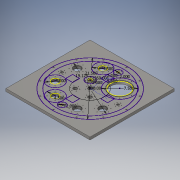
# Autodesk Inventor part: Top Plate
Saved by Autodesk Inventor 2018 (Build 220112000, 112)
## iProperties
Created: 2018-08-07
Part Number: Top Plate
Material: Stainless Steel, Austenitic
Document SubType Name: Modeling
Designer: freyja
Density: 8 g/cm^3
Appearance: Semi-Polished
Mass: 52241 g
Surface Area: 7917.75 cm^2
Volume: 6530.12 cm^3
Author: freyja
Autodesk Inventor part; units mm, degrees
ref_plane "YZ Plane" through (0, 0, 0) normal (1, 0, 0) x (0, 1, 0)
ref_plane "XZ Plane" through (0, 0, 0) normal (0, 1, 0) x (-1, 0, 0)
ref_plane "XY Plane" through (0, 0, 0) normal (0, 0, 1) x (1, 0, 0)
sketch "Sketch1" plane through (0, 0, 0) normal (0, 1, 0) x (-1, 0, 0)
  line L0 (304.8, 304.8) -> (-304.8, 304.8)
  line L1 (-304.8, 304.8) -> (-304.8, -304.8)
  line L2 (-304.8, -304.8) -> (304.8, -304.8)
  line L3 (304.8, -304.8) -> (304.8, 304.8)
  line L4 (304.8, 304.8) -> (-304.8, -304.8) construction
  line L5 (-304.8, 304.8) -> (304.8, -304.8) construction
  point P0 (0, 0)
  dimension "d0" = 609.6
  dimension "d1" = 609.6
  constraints: 12 end point, 2 midpoint, 2 parallel, 1 horizontal, 1 perpendicular
  measures "d0" distance of L2.end L1.end
  measures "d1" distance of L1.end L0.end
extrude "Extrusion1" add sketch "Sketch1" along normal blind 19.05
sketch "Sketch23" plane through (0, 19.05, 0) normal (0, 1, 0) x (1, 0, 0)
  circle A0 centre (0, 0) radius 273.05
  circle A1 centre (0, 0) radius 242.8875
  dimension "d167" = 546.1
  dimension "d168" = 485.775
  constraints: 2 centre point, 2 coincident
  measures "d167" diameter of A0
  measures "d168" diameter of A1
sketch "Sketch2" plane through (0, 19.05, 0) normal (0, 1, 0) x (1, 0, 0)
  line L0 (0, 0) -> (107.7631, 107.7631) construction
  line L1 (0, 0) -> (152.4, 0) construction
  circle A0 centre (107.7631, 107.7631) radius 118.745 construction
  circle A1 centre (107.7631, 107.7631) radius 66.675
  dimension "d4" = 152.4
  dimension "d5" = 45
  dimension "d6" = 237.49
  dimension "d7" = 133.35
  constraints: 4 end point, 2 centre point, 2 coincident, 1 equal length, 1 horizontal
  measures "d4" distance of L0.start L0.end
  measures "d5" angle of L1 L0
  measures "d6" diameter of A0
  measures "d7" diameter of A1
extrude "Extrusion2" cut sketch "Sketch2" against normal up to surface (19.05 mm away)
sketch "Sketch3" plane through (0, 19.05, 0) normal (0, 1, 0) x (1, 0, 0)
  circle A0 centre (107.7631, 107.7631) radius 66.675 projected
  line L0 (107.7631, 107.7631) -> (194.1231, 107.7631) construction
  line L1 (107.7631, 107.7631) -> (194.1231, 107.7631) construction
  line L2 (107.7631, 107.7631) -> (168.8288, 168.8288) construction
  line L3 (107.7631, 107.7631) -> (107.7631, 194.1231) construction
  line L4 (107.7631, 107.7631) -> (46.6973, 168.8288) construction
  line L5 (107.7631, 107.7631) -> (21.4031, 107.7631) construction
  line L6 (107.7631, 107.7631) -> (46.6973, 46.6973) construction
  line L7 (107.7631, 107.7631) -> (107.7631, 21.4031) construction
  line L8 (107.7631, 107.7631) -> (168.8288, 46.6973) construction
  point P0 (0, 0)
  dimension "d10" = 86.36
  dimension "d11" = 0
  dimension "d14" = 360
  constraints: 18 end point, 2 coincident, 2 horizontal, 1 collinear, 23 other
  measures "d10" distance of L0.start L0.end
  measures "d11" distance between parallel lines of L0 L1
hole "Hole1" at (194.1231, 19.05, -107.7631) at (168.8288, 19.05, -168.8288) at (107.7631, 19.05, -194.1231) at (46.6973, 19.05, -168.8288) at (21.4031, 19.05, -107.7631) at (46.6973, 19.05, -46.6973) at (107.7631, 19.05, -21.4031) at (168.8288, 19.05, -46.6973) direction (0, -1, 0) diameter 4.9784 depth 15.24 tip angle 118 thread size "1/4-20 UNC" class "2B" standard "ANSI Unified Screw Threads"
sketch "Sketch4" plane through (0, 19.05, 0) normal (0, 1, 0) x (1, 0, 0)
  line L0 (0, 0) -> (-172.6516, -80.5088) construction
  line L1 (0, 0) -> (190.5, 0) construction
  circle A0 centre (-172.6516, -80.5088) radius 26.289
  dimension "d23" = 190.5
  dimension "d24" = 205
  dimension "d25" = 52.578
  constraints: 4 end point, 1 centre point, 1 coincident, 1 equal length, 1 horizontal
  measures "d23" distance of L0.start L0.end
  measures "d25" diameter of A0
extrude "Extrusion3" cut sketch "Sketch4" against normal blind 2.54
sketch "Sketch5" plane through (-172.6516, 16.51, 80.5088) normal (0, 1, 0) x (1, 0, 0)
  circle A0 centre (0, 0) radius 26.289 projected
  circle A1 centre (0, 0) radius 24.13
  point P0 (172.6516, 80.5088)
  dimension "d28" = 48.26
  constraints: 1 centre point, 1 coincident
  measures "d28" diameter of A1
extrude "Extrusion4" cut sketch "Sketch5" against normal up to surface (16.51 mm away) contours A1
sketch "Sketch6" plane through (0, 19.05, 0) normal (0, 1, 0) x (1, 0, 0)
  circle A0 centre (-172.6516, -80.5088) radius 24.13 construction
  line L0 (-172.6516, -80.5088) -> (-131.3766, -80.5088) construction
  line L1 (-172.6516, -80.5088) -> (-131.3766, -80.5088) construction
  line L2 (-172.6516, -80.5088) -> (-143.4658, -51.3229) construction
  line L3 (-172.6516, -80.5088) -> (-172.6516, -39.2338) construction
  line L4 (-172.6516, -80.5088) -> (-201.8375, -51.3229) construction
  line L5 (-172.6516, -80.5088) -> (-213.9266, -80.5088) construction
  line L6 (-172.6516, -80.5088) -> (-201.8375, -109.6946) construction
  line L7 (-172.6516, -80.5088) -> (-172.6516, -121.7838) construction
  line L8 (-172.6516, -80.5088) -> (-143.4658, -109.6946) construction
  point P0 (0, 0)
  dimension "d31" = 41.275
  dimension "d32" = 0
  dimension "d35" = 360
  constraints: 18 end point, 2 coincident, 2 horizontal, 1 collinear, 23 other
  measures "d31" distance of L0.start L0.end
  measures "d32" distance between parallel lines of L0 L1
hole "Hole2" at (-143.4658, 19.05, 51.3229) at (-172.6516, 19.05, 39.2338) at (-201.8375, 19.05, 51.3229) at (-213.9266, 19.05, 80.5088) at (-201.8375, 19.05, 109.6946) at (-172.6516, 19.05, 121.7838) at (-143.4658, 19.05, 109.6946) at (-131.3766, 19.05, 80.5088) direction (0, -1, 0) diameter 3.9624 depth 13.6144 tip angle 118 thread size "10-32 UNF" class "2B" standard "ANSI Unified Screw Threads"
pattern_circular "Circular Pattern1" count 3 over 180 about axis through (0, -10, 0) along (0, 1, 0) of "Extrusion4", "Extrusion3", "Hole2" both ways yes
sketch "Sketch7" plane through (0, 19.05, 0) normal (0, 1, 0) x (1, 0, 0)
  line L0 (0, 0) -> (-53.8815, 53.8815) construction
  line L1 (0, 0) -> (76.2, 0) construction
  circle A0 centre (-53.8815, 53.8815) radius 13.208
  dimension "d44" = 76.2
  dimension "d45" = 135
  dimension "d46" = 26.416
  constraints: 4 end point, 1 centre point, 1 coincident, 1 equal length, 1 horizontal
  measures "d44" distance of L0.start L0.end
  measures "d45" angle of L1 L0
  measures "d46" diameter of A0
extrude "Extrusion5" cut sketch "Sketch7" against normal blind 2.54
sketch "Sketch8" plane through (0, 19.05, 0) normal (0, 1, 0) x (1, 0, 0)
  circle A0 centre (-53.8815, 53.8815) radius 13.208 projected
  circle A1 centre (-53.8815, 53.8815) radius 11.43
  point P0 (0, 0)
  dimension "d49" = 22.86
  constraints: 1 centre point, 1 coincident
  measures "d49" diameter of A1
extrude "Extrusion6" cut sketch "Sketch8" against normal up to surface (19.05 mm away) contours A1
sketch "Sketch9" plane through (0, 19.05, 0) normal (0, 1, 0) x (1, 0, 0)
  circle A0 centre (-53.8815, 53.8815) radius 13.208 projected
  line L0 (-53.8815, 53.8815) -> (-29.8785, 53.8815) construction
  line L1 (-53.8815, 53.8815) -> (-29.8785, 53.8815) construction
  line L2 (-53.8815, 53.8815) -> (-41.88, 74.6687) construction
  line L3 (-53.8815, 53.8815) -> (-65.883, 74.6687) construction
  line L4 (-53.8815, 53.8815) -> (-77.8845, 53.8815) construction
  line L5 (-53.8815, 53.8815) -> (-65.883, 33.0943) construction
  line L6 (-53.8815, 53.8815) -> (-41.88, 33.0943) construction
  point P0 (0, 0)
  dimension "d52" = 24.003
  dimension "d53" = 0
  dimension "d56" = 360
  constraints: 14 end point, 2 coincident, 2 horizontal, 1 collinear, 17 other
  measures "d52" distance of L0.start L0.end
  measures "d53" distance between parallel lines of L0 L1
hole "Hole3" at (-29.8785, 19.05, -53.8815) at (-41.88, 19.05, -74.6687) at (-65.883, 19.05, -74.6687) at (-77.8845, 19.05, -53.8815) at (-65.883, 19.05, -33.0943) at (-41.88, 19.05, -33.0943) direction (0, -1, 0) diameter 3.9624 depth 13.6144 tip angle 118 thread size "10-32 UNF" class "2B" standard "ANSI Unified Screw Threads"
pattern_circular "Circular Pattern5" count 3 over 180 about axis through (0, -10, 0) along (0, 1, 0) of "Extrusion5", "Extrusion6", "Hole3"
sketch "Sketch26" plane through (0, 19.05, 0) normal (0, 1, 0) x (1, 0, 0)
  line L0 (0, 0) -> (0, 203.2) construction
  line L1 (0, 0) -> (203.2, 0) construction
  circle A0 centre (0, 203.2) radius 8.636
  dimension "d185" = 203.2
  dimension "d186" = 270
  dimension "d187" = 17.272
  constraints: 4 end point, 1 centre point, 1 coincident, 1 horizontal, 1 perpendicular
  measures "d185" distance of L0.start L0.end
  measures "d187" diameter of A0
extrude "Extrusion16" cut sketch "Sketch26" against normal blind 2.54
sketch "Sketch27" plane through (0, 19.05, 0) normal (0, 1, 0) x (1, 0, 0)
  circle A0 centre (0, 203.2) radius 8.636 projected
  circle A1 centre (0, 203.2) radius 6.35
  point P0 (0, 0)
  dimension "d190" = 12.7
  constraints: 1 centre point, 1 coincident
  measures "d190" diameter of A1
extrude "Extrusion17" cut sketch "Sketch27" against normal up to surface (19.05 mm away) contours A1
sketch "Sketch28" plane through (0, 19.05, 0) normal (0, 1, 0) x (1, 0, 0)
  circle A0 centre (0, 203.2) radius 8.636 projected
  line L0 (0, 203.2) -> (-19.05, 203.2) construction
  line L1 (0, 203.2) -> (19.05, 203.2) construction
  line L2 (0, 203.2) -> (-9.525, 186.7022) construction
  line L3 (0, 203.2) -> (9.525, 186.7022) construction
  line L4 (0, 203.2) -> (19.05, 203.2) construction
  line L5 (0, 203.2) -> (9.525, 219.6978) construction
  line L6 (0, 203.2) -> (-9.525, 219.6978) construction
  point P0 (0, 0)
  dimension "d193" = 19.05
  dimension "d194" = 180
  dimension "d204" = 360
  constraints: 14 end point, 2 coincident, 2 horizontal, 1 collinear, 17 other
  measures "d193" distance of L0.start L0.end
  measures "d194" angle of L0 L1
hole "Hole9" at (-19.05, 19.05, -203.2) at (-9.525, 19.05, -219.6978) at (9.525, 19.05, -219.6978) at (19.05, 19.05, -203.2) at (9.525, 19.05, -186.7022) at (-9.525, 19.05, -186.7022) direction (0, -1, 0) diameter 3.9624 depth 13.6144 tip angle 118 thread size "10-32 UNF" class "2B" standard "ANSI Unified Screw Threads"
pattern_circular "Circular Pattern6" count 4 over 360 about axis through (0, -10, 0) along (0, 1, 0) of "Extrusion16", "Extrusion17", "Hole9"
sketch "Sketch29" plane through (0, 19.05, 0) normal (0, 1, 0) x (1, 0, 0)
  line L0 (0, 0) -> (0, 127) construction
  line L1 (0, 0) -> (127, 0) construction
  line L2 (-25.4, 101.6) -> (25.4, 101.6)
  line L3 (25.4, 101.6) -> (25.4, 152.4)
  line L4 (25.4, 152.4) -> (-25.4, 152.4)
  line L5 (-25.4, 152.4) -> (-25.4, 101.6)
  line L6 (-25.4, 101.6) -> (25.4, 152.4) construction
  line L7 (25.4, 101.6) -> (-25.4, 152.4) construction
  line L8 (-101.6, -25.4) -> (-101.6, 25.4)
  line L9 (-152.4, -25.4) -> (-101.6, -25.4)
  line L10 (-101.6, 25.4) -> (-152.4, 25.4)
  line L11 (-152.4, 25.4) -> (-152.4, -25.4)
  line L12 (25.4, -101.6) -> (-25.4, -101.6)
  line L13 (25.4, -152.4) -> (25.4, -101.6)
  line L14 (-25.4, -101.6) -> (-25.4, -152.4)
  line L15 (-25.4, -152.4) -> (25.4, -152.4)
  line L16 (101.6, 25.4) -> (101.6, -25.4)
  line L17 (152.4, 25.4) -> (101.6, 25.4)
  line L18 (101.6, -25.4) -> (152.4, -25.4)
  line L19 (152.4, -25.4) -> (152.4, 25.4)
  dimension "d213" = 127
  dimension "d214" = 90
  dimension "d215" = 50.8
  dimension "d216" = 50.8
  dimension "d219" = 360
  constraints: 40 end point, 2 horizontal, 2 midpoint, 2 parallel, 2 perpendicular, 33 other
  measures "d213" distance of L0.start L0.end
  measures "d214" angle of L1 L0
  measures "d215" distance of L4.end L3.end
  measures "d216" distance of L3.end L2.end
sketch "Sketch30" plane through (0, 19.05, 0) normal (0, 1, 0) x (1, 0, 0)
  line L0 (0, 0) -> (-80.5088, -172.6516) construction
  line L1 (0, 0) -> (190.5, 0) construction
  circle A0 centre (-80.5088, -172.6516) radius 26.289
  dimension "d221" = 190.5
  dimension "d222" = 115
  dimension "d223" = 52.578
  constraints: 4 end point, 1 centre point, 1 coincident, 1 equal length, 1 horizontal
  measures "d221" distance of L0.start L0.end
  measures "d222" angle of L0 L1
  measures "d223" diameter of A0
extrude "Extrusion18" cut sketch "Sketch30" against normal blind 2.54
sketch "Sketch31" plane through (0, 19.05, 0) normal (0, 1, 0) x (1, 0, 0)
  circle A0 centre (-80.5088, -172.6516) radius 26.289 projected
  circle A1 centre (-80.5088, -172.6516) radius 24.13
  point P0 (0, 0)
  dimension "d226" = 48.26
  constraints: 1 centre point, 1 coincident
  measures "d226" diameter of A1
extrude "Extrusion19" cut sketch "Sketch31" against normal up to surface (19.05 mm away) contours A1
sketch "Sketch32" plane through (0, 19.05, 0) normal (0, 1, 0) x (1, 0, 0)
  circle A0 centre (-80.5088, -172.6516) radius 26.289 construction
  line L0 (-80.5088, -172.6516) -> (-121.7838, -172.6516) construction
  line L1 (-80.5088, -172.6516) -> (-109.6946, -201.8375) construction
  line L2 (-80.5088, -172.6516) -> (-80.5088, -213.9266) construction
  line L3 (-80.5088, -172.6516) -> (-51.3229, -201.8375) construction
  line L4 (-80.5088, -172.6516) -> (-39.2338, -172.6516) construction
  line L5 (-80.5088, -172.6516) -> (-51.3229, -143.4658) construction
  line L6 (-80.5088, -172.6516) -> (-80.5088, -131.3766) construction
  line L7 (-80.5088, -172.6516) -> (-109.6946, -143.4658) construction
  point P0 (0, 0)
  dimension "d229" = 41.275
  dimension "d232" = 360
  constraints: 16 end point, 2 coincident, 1 horizontal, 23 other
  measures "d229" distance of L0.start L0.end
hole "Hole10" at (-109.6946, 19.05, 143.4658) at (-121.7838, 19.05, 172.6516) at (-80.5088, 19.05, 131.3766) at (-51.3229, 19.05, 143.4658) at (-39.2338, 19.05, 172.6516) at (-51.3229, 19.05, 201.8375) at (-80.5088, 19.05, 213.9266) at (-109.6946, 19.05, 201.8375) direction (0, -1, 0) diameter 3.9624 depth 13.6144 tip angle 118 thread size "10-32 UNF" class "2B" standard "ANSI Unified Screw Threads"
sketch "Sketch25" plane through (0, 19.05, 0) normal (0, 1, 0) x (1, 0, 0)
  circle A0 centre (-172.6516, -80.5088) radius 26.289 projected
  circle A1 centre (-172.6516, -80.5088) radius 57.15
  circle A2 centre (107.7631, 107.7631) radius 66.675 projected
  circle A3 centre (107.7631, 107.7631) radius 95.25
  circle A4 centre (-53.8815, 53.8815) radius 11.43 projected
  circle A5 centre (-53.8815, 53.8815) radius 31.75
  circle A6 centre (0, 203.2) radius 6.35 projected
  circle A7 centre (0, 203.2) radius 25.4
  circle A8 centre (-80.5088, -172.6516) radius 24.13 projected
  circle A9 centre (-80.5088, -172.6516) radius 57.15
  circle A10 centre (0, -203.2) radius 6.35 projected
  circle A11 centre (0, -203.2) radius 25.4
  circle A12 centre (-80.5088, 172.6516) radius 24.13 projected
  circle A13 centre (-80.5088, 172.6516) radius 57.15
  point P0 (0, 0)
  dimension "d206" = 114.3
  dimension "d207" = 190.5
  dimension "d208" = 63.5
  dimension "d209" = 50.8
  dimension "d241" = 114.3
  dimension "d245" = 50.8
  dimension "d246" = 114.3
  constraints: 7 centre point, 7 coincident
  measures "d206" diameter of A1
  measures "d207" diameter of A3
  measures "d208" diameter of A5
  measures "d209" diameter of A7
  measures "d241" diameter of A9
  measures "d245" diameter of A11
  measures "d246" diameter of A13
pattern_circular "Circular Pattern7" count 3 over 180 about axis through (0, -10, 0) along (0, 1, 0) of "Extrusion18", "Extrusion19", "Hole10" both ways yes
sketch "Sketch33" plane through (0, 19.05, 0) normal (0, 1, 0) x (1, 0, 0)
  circle A0 centre (0, 0) radius 13.208
  dimension "d247" = 26.416
  constraints: 1 centre point, 1 coincident
  measures "d247" diameter of A0
extrude "Extrusion20" cut sketch "Sketch33" against normal blind 2.54
sketch "Sketch34" plane through (0, 19.05, 0) normal (0, 1, 0) x (1, 0, 0)
  circle A0 centre (0, 0) radius 13.208 projected
  circle A1 centre (0, 0) radius 11.43
  dimension "d250" = 22.86
  constraints: 1 centre point, 1 coincident
  measures "d250" diameter of A1
extrude "Extrusion21" cut sketch "Sketch34" against normal up to surface (19.05 mm away) contours A1
sketch "Sketch35" plane through (0, 19.05, 0) normal (0, 1, 0) x (1, 0, 0)
  line L0 (0, 0) -> (-24.003, 0) construction
  line L1 (0, 0) -> (-12.0015, -20.7872) construction
  line L2 (0, 0) -> (12.0015, -20.7872) construction
  line L3 (0, 0) -> (24.003, 0) construction
  line L4 (0, 0) -> (12.0015, 20.7872) construction
  line L5 (0, 0) -> (-12.0015, 20.7872) construction
  dimension "d253" = 24.003
  dimension "d256" = 360
  constraints: 12 end point, 2 coincident, 1 horizontal, 17 other
  measures "d253" distance of L0.start L0.end
hole "Hole11" at (12.0015, 19.05, -20.7872) at (-12.0015, 19.05, -20.7872) at (-24.003, 19.05, 0) at (-12.0015, 19.05, 20.7872) at (12.0015, 19.05, 20.7872) at (24.003, 19.05, 0) direction (0, -1, 0) diameter 3.9624 depth 13.6144 tip angle 118 thread size "10-32 UNF" class "2B" standard "ANSI Unified Screw Threads"
sketch "Sketch37" plane through (0, 19.05, 0) normal (0, 1, 0) x (1, 0, 0)
  line L0 (0, 0) -> (-264.16, 0)
  dimension "d277" = 264.16
  constraints: 2 end point, 1 horizontal
  measures "d277" distance of L0.start L0.end
hole "Hole13" at (-264.16, 19.05, 0) direction (0, -1, 0) diameter 8.9916 depth 21.1074 tip angle 118 clearance for "Socket Head Cap Screw" size "M8" standard "Ansi Metric M Profile"
pattern_circular "Circular Pattern9" count 12 over 360 about axis through (0, -10, 0) along (0, 1, 0) of "Hole13"
sketch "Sketch38" plane through (0, 19.05, 0) normal (0, 1, 0) x (1, 0, 0)
  circle A0 centre (107.7631, 107.7631) radius 66.675 projected
  circle A1 centre (107.7631, 107.7631) radius 71.12
  circle A2 centre (107.7631, 107.7631) radius 74.295
  point P0 (0, 0)
  dimension "d288" = 142.24
  dimension "d289" = 148.59
  constraints: 2 centre point, 2 coincident
  measures "d288" diameter of A1
  measures "d289" diameter of A2
extrude "Extrusion22" cut sketch "Sketch38" against normal blind 3.175 contours A2
body "Solid1"
